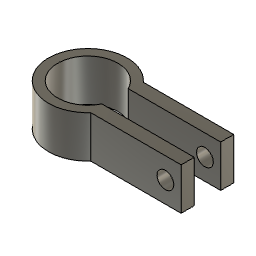
uchyt_kruh (Autodesk Fusion 360 design; units mm, degrees)
Autodesk Fusion 360 part; units mm, degrees
sketch "Sketch3" plane through (0, 0, 0) normal (0, 0, 1) x (1, 0, 0)
  line L0 (0, 0) -> (7.5, 0)
  line L1 (5.5732, 5.0189) -> (22.806, 5.0189)
  line L2 (22.806, 5.0189) -> (22.806, 2.5189)
  line L3 (22.806, 2.5189) -> (5.1689, 2.5189)
  line L4 (5.5732, -5.0189) -> (22.806, -5.0189)
  line L5 (22.806, -2.5189) -> (5.1689, -2.5189)
  line L6 (22.806, -5.0189) -> (22.806, -2.5189)
  arc A0 (5.1689, 2.5189) -> (5.1689, -2.5189) centre (0, 0) ccw
  arc A1 (7.0644, 2.5189) -> (7.0644, -2.5189) centre (0, 0) ccw
  dimension "d8" = 11.5
  dimension "d9" = 15
  dimension "d12" = 2.5
  constraint coincident L0.start A0.centre
  constraint concentric A0 A1
  constraint horizontal L0
  constraint horizontal L1
  constraint perpendicular L1 L2
  constraint perpendicular L2 L3
  constraint symmetric L0 L1.end L4.end
  constraint symmetric L0 L2.end L5.start
  constraint symmetric L0 L3.end L5.end
  constraint coincident L3 A1.start
  constraint coincident L5 A1.end
  constraint coincident A1 L4.start
  constraint coincident A1 L1.start
  measures "d8" diameter of A0
  measures "d9" diameter of A1
  measures "d12" distance of L1.end L2.end
extrude "Extrude3" add sketch "Sketch3" along normal blind 8
sketch "Sketch5" plane through (0, 5.0189, 0) normal (0, 1, 0) x (-1, 0, 0)
  line L0 (-22.806, 0) -> (-5.5732, 0)
  line L1 (-5.5732, 0) -> (-5.5732, 8)
  line L2 (-5.5732, 8) -> (-22.806, 8)
  line L3 (-22.806, 8) -> (-22.806, 0)
  line L4 (-22.806, 4) -> (-19.806, 4)
  circle A0 centre (-19.806, 4) radius 1.6
  dimension "d15" = 3
  dimension "d16" = 3.2
  constraint midpoint L3 L4.start
  constraint perpendicular L3 L4
  constraint coincident L4.end A0.centre
  measures "d15" distance of L4.start L4.end
  measures "d16" diameter of A0
extrude "Extrude4" cut sketch "Sketch5" against normal blind 14 contours A0
